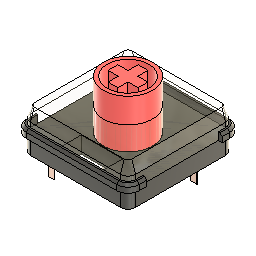
Choc v2 v34 (Autodesk Fusion 360 design; units mm, degrees)
Autodesk Fusion 360 part; units mm, degrees
note: some values were not read from the file. Chosen so that the rebuilt part matches the saved one: which face or edge a step refers to; a side; which pieces of a blend or face edit are solid. Set by a fixed rule: which sketch regions a step uses.
sketch "Base" plane through (0, 0, 0) normal (0, 0, 1) x (1, 0, 0)
  line L0 (6, 7.5) -> (-6, 7.5)
  line L1 (-7.5, 6) -> (-7.5, -6)
  line L2 (-6, -7.5) -> (6, -7.5)
  line L3 (7.5, -6) -> (7.5, 6)
  line L4 (7.5, 7.5) -> (-7.5, -7.5) construction
  line L5 (-7.5, 7.5) -> (7.5, -7.5) construction
  line L6 (-9, 5) -> (9, 5)
  line L7 (20, 0) -> (2.5, 0)
  line L8 (-9, -5) -> (9, -5)
  line L9 (5.975, 6.975) -> (-5.975, 6.975)
  line L10 (-6.975, 5.975) -> (-6.975, -5.975)
  line L11 (-5.975, -6.975) -> (5.975, -6.975)
  line L12 (6.975, -5.975) -> (6.975, 5.975)
  line L13 (6.975, 6.975) -> (-6.975, -6.975) construction
  line L14 (-6.975, 6.975) -> (6.975, -6.975) construction
  arc A0 (7.5, 6) -> (6, 7.5) centre (6, 6) ccw
  arc A1 (6, -7.5) -> (7.5, -6) centre (6, -6) ccw
  arc A2 (-7.5, -6) -> (-6, -7.5) centre (-6, -6) ccw
  arc A3 (-6, 7.5) -> (-7.5, 6) centre (-6, 6) ccw
  arc A4 (6.975, 5.975) -> (5.975, 6.975) centre (5.975, 5.975) ccw
  arc A5 (5.975, -6.975) -> (6.975, -5.975) centre (5.975, -5.975) ccw
  arc A6 (-6.975, -5.975) -> (-5.975, -6.975) centre (-5.975, -5.975) ccw
  arc A7 (-5.975, 6.975) -> (-6.975, 5.975) centre (-5.975, 5.975) ccw
  circle A8 centre (0, 0) radius 3.25
  circle A9 centre (0, 0) radius 2.4
  line L15 (2.75, -3.455) -> (-2.75, -3.455)
  line L16 (-2.75, -3.455) -> (-2.75, -6.405)
  line L17 (-2.75, -6.405) -> (2.75, -6.405)
  line L18 (2.75, -6.405) -> (2.75, -3.455)
  line L19 (2.75, -3.455) -> (-2.75, -6.405) construction
  line L20 (-2.75, -3.455) -> (2.75, -6.405) construction
  line L21 (0, 1.75) -> (0, 22.5)
  line L22 (2, 0.65) -> (-2, 0.65)
  line L23 (-2, 0.65) -> (-2, -0.65)
  line L24 (-2, -0.65) -> (2, -0.65)
  line L25 (2, -0.65) -> (2, 0.65)
  line L26 (2, 0.65) -> (-2, -0.65) construction
  line L27 (-2, 0.65) -> (2, -0.65) construction
  line L28 (0.65, 2) -> (0.65, -2)
  line L29 (-0.65, 2) -> (0.65, 2)
  line L30 (-0.65, -2) -> (-0.65, 2)
  line L31 (0.65, -2) -> (-0.65, -2)
  line L32 (-4.6, -5.1) -> (-5.4, -5.1)
  line L33 (-5.4, -5.1) -> (-5.4, -5.2)
  line L34 (-5.4, -5.2) -> (-4.6, -5.2)
  line L35 (-4.6, -5.2) -> (-4.6, -5.1)
  line L36 (-4.6, -5.1) -> (-5.4, -5.2) construction
  line L37 (-5.4, -5.1) -> (-4.6, -5.2) construction
  line L38 (1.75, 0) -> (22.5, 0)
  line L39 (0.4, 5.95) -> (-0.4, 5.95)
  line L40 (-0.4, 5.95) -> (-0.4, 5.85)
  line L41 (-0.4, 5.85) -> (0.4, 5.85)
  line L42 (0.4, 5.85) -> (0.4, 5.95)
  line L43 (0.4, 5.95) -> (-0.4, 5.85) construction
  line L44 (-0.4, 5.95) -> (0.4, 5.85) construction
  line L45 (5.4, 3.85) -> (4.6, 3.85)
  line L46 (4.6, 3.85) -> (4.6, 3.75)
  line L47 (4.6, 3.75) -> (5.4, 3.75)
  line L48 (5.4, 3.75) -> (5.4, 3.85)
  line L49 (5.4, 3.85) -> (4.6, 3.75) construction
  line L50 (4.6, 3.85) -> (5.4, 3.75) construction
  line L51 (9.9048, 2.5) -> (-9, 2.5)
  line L52 (9.9048, -2.5) -> (-9, -2.5)
  circle A10 centre (-5, -5.15) radius 0.7
  line L53 (-5, -5.85) -> (-3.3, -5.85)
  line L54 (-3.3, -5.85) -> (-3.3, -3.5282)
  line L55 (-3.3, -3.5282) -> (-5.7, -3.5282)
  line L56 (-5.7, -3.5282) -> (-5.7, -5.15)
  arc A11 (-5.7, -5.15) -> (-5, -5.85) centre (-5, -5.15) ccw
  line L57 (6, -7.5) -> (7.5, -7.5)
  line L58 (7.5, -6) -> (7.5, -7.5)
  line L59 (7.5, 6) -> (7.5, 7.5)
  line L60 (6, 7.5) -> (7.5, 7.5)
  line L61 (-6, 7.5) -> (-7.5, 7.5)
  line L62 (-7.5, 6) -> (-7.5, 7.5)
  line L63 (-7.5, -6) -> (-7.5, -7.5)
  line L64 (-6, -7.5) -> (-7.5, -7.5)
  line L65 (7.5, -2.5) -> (7.5, 2.5)
  line L66 (7.5, 2.5) -> (8.975, 2.5)
  line L67 (8.975, 2.5) -> (8.975, -2.5)
  line L68 (8.975, -2.5) -> (7.5, -2.5)
  line L69 (-7.5, -2.5) -> (-7.5, 2.5)
  line L70 (-7.5, 2.5) -> (-8.975, 2.5)
  line L71 (-8.975, 2.5) -> (-8.975, -2.5)
  line L72 (-8.975, -2.5) -> (-7.5, -2.5)
  point P0 (0, -4.93)
  point P1 (-5, -5.15)
  point P2 (0, 5.9)
  point P3 (5, 3.8)
  point P4 (-5, -5.15)
  dimension "d1" = 15
  dimension "d2" = 10
  dimension "d3" = 13.95
  dimension "d4" = 1.5
  dimension "d5" = 1
  dimension "d6" = 6.5
  dimension "d7" = 4.8
  dimension "d25" = 4.93
  dimension "d26" = 2.95
  dimension "d27" = 5.5
  dimension "d30" = 4
  dimension "d31" = 1.3
  dimension "d34" = 5.15
  dimension "d35" = 5
  dimension "d36" = 0.8
  dimension "d37" = 0.1
  dimension "d41" = 0.1
  dimension "d42" = 0.8
  dimension "d43" = 5.9
  dimension "d44" = 0.1
  dimension "d45" = 0.8
  dimension "d46" = 5
  dimension "d47" = 3.8
  dimension "d54" = 5
  dimension "d58" = 1.4
  dimension "d74" = 0.7
  dimension "d91" = 2
  dimension "d92" = 2
  constraint horizontal L0
  constraint perpendicular L0 L1
  constraint parallel L0 L2
  constraint parallel L1 L3
  constraint coincident L4 A8.centre
  constraint coincident L5 A8.centre
  constraint coincident A8.centre A9.centre
  constraint perpendicular L3 L6
  constraint symmetric L6.start L7 L8.start
  constraint symmetric L6.end L7 L8.end
  constraint horizontal L9
  constraint perpendicular L9 L10
  constraint parallel L9 L11
  constraint parallel L10 L12
  constraint coincident L4 L13.start
  constraint coincident L13 A8.centre
  constraint coincident L14 A8.centre
  constraint coincident L4.start L0
  constraint coincident L4.start L3
  constraint tangent L0 A0
  constraint tangent L3 A0
  constraint coincident L5.end L3
  constraint coincident L5.end L2
  constraint tangent L3 A1
  constraint tangent L2 A1
  constraint equal A0 A1
  constraint coincident L4.end L2
  constraint coincident L4.end L1
  constraint tangent L2 A2
  constraint tangent L1 A2
  constraint equal A0 A2
  constraint coincident L5.start L1
  constraint coincident L5.start L0
  constraint tangent L1 A3
  constraint tangent L0 A3
  constraint equal A0 A3
  constraint equal L0 L1
  constraint coincident L13.start L9
  constraint coincident L13.start L12
  constraint tangent L9 A4
  constraint tangent L12 A4
  constraint coincident L14.end L12
  constraint coincident L14.end L11
  constraint tangent L12 A5
  constraint tangent L11 A5
  constraint equal A4 A5
  constraint coincident L13.end L11
  constraint coincident L13.end L10
  constraint tangent L11 A6
  constraint tangent L10 A6
  constraint equal A4 A6
  constraint coincident L14.start L10
  constraint coincident L14.start L9
  constraint tangent L10 A7
  constraint tangent L9 A7
  constraint equal A4 A7
  constraint horizontal L15
  constraint perpendicular L15 L16
  constraint parallel L15 L17
  constraint parallel L16 L18
  constraint coincident L19 P0
  constraint coincident L20 P0
  constraint coincident P0 L21
  constraint horizontal L22
  constraint perpendicular L22 L23
  constraint parallel L22 L24
  constraint parallel L23 L25
  constraint coincident L26 A8.centre
  constraint coincident L27 A8.centre
  constraint symmetric L4 L22.start L28.start
  constraint symmetric L4 L22.end L28.end
  constraint symmetric L4 L23.end L30.start
  constraint symmetric L4 L24.end L29.start
  constraint horizontal L32
  constraint perpendicular L32 L33
  constraint parallel L32 L34
  constraint parallel L33 L35
  constraint coincident L36 P4
  constraint coincident L37 P4
  constraint horizontal L39
  constraint perpendicular L39 L40
  constraint parallel L39 L41
  constraint parallel L40 L42
  constraint coincident L43 P2
  constraint coincident L44 P2
  constraint coincident L21 P2
  constraint horizontal L45
  constraint perpendicular L45 L46
  constraint parallel L45 L47
  constraint parallel L46 L48
  constraint coincident L49 P3
  constraint coincident L50 P3
  constraint perpendicular L1 L51
  constraint symmetric L7 L51.start L52.start
  constraint symmetric L7 L51.end L52.end
  constraint coincident P4 P1
  constraint horizontal L53
  constraint perpendicular L53 L54
  constraint tangent L53 A11
  constraint tangent L56 A11
  constraint tangent A1 L57
  constraint tangent A0 L59
  constraint tangent A0 L60
  constraint perpendicular L65 L66
  constraint parallel L65 L67
  constraint parallel L66 L68
  constraint coincident L3 L65.end
  constraint coincident L51 L65.end
  constraint perpendicular L51 L65
  constraint coincident L52 L65.start
  constraint perpendicular L69 L70
  constraint parallel L69 L71
  constraint parallel L70 L72
  constraint coincident L1 L69.end
  constraint coincident L51 L69.end
  constraint perpendicular L51 L69
  constraint coincident L52 L69.start
  measures "d1" distance of L1 L3
  measures "d2" distance of L6 L8
  measures "d3" distance of L10 L12
  measures "d4" radius of A0
  measures "d5" radius of A4
  measures "d6" diameter of A8
  measures "d7" diameter of A9
  measures "d25" distance of A8.centre P0
  measures "d26" distance of L15 L17
  measures "d27" distance of L16 L18
  measures "d30" distance of L23 L25
  measures "d31" distance of L22 L24
  measures "d34" distance of P4 L38
  measures "d35" distance of L21 P4
  measures "d36" distance of L33 L35
  measures "d37" distance of L32 L34
  measures "d41" distance of L39 L41
  measures "d42" distance of L40 L42
  measures "d43" distance of A8.centre P2
  measures "d44" distance of L45 L47
  measures "d45" distance of L46 L48
  measures "d46" distance of L21 P3
  measures "d47" distance of L38 P3
  measures "d54" distance of L51 L52
  measures "d58" diameter of A10
  measures "d74" radius of A11
  measures "d91" distance of L12 L67
  measures "d92" distance of L10 L71
extrude "Extrude1" add sketch "Base" along normal blind 3.1 contours L6 L9 L10 A7 L21 L39 L40 L41 | L6 L9 L12 A4 L21 L39 L41 L42 | L21 L39 L41 L42 | L21 L39 L40 L41 | L6 L12 A8 L21 L51 | L7 L12 A8 L38 L51 | L6 L10 A8 L21 L51 | L7 L12 A8 L38 L52 | L10 A8 L51 L52 | L8 L10 L12 A8 L15 L16 L18 L52 L54 L55 L56 | L8 L10 L11 L12 A5 A6 L16 L17 L18 A10 L53 L54 L56 A11 | L8 L16 L17 L18 | L8 L15 L16 L18 | L8 A10 L54 L55 L56 | L8 A10 L56 | L8 A10 | L8 A10 A11 | L8 A10 L53 L54 | L32 L33 L34 L35 | L45 L46 L47 L48 makes body 1
chamfer "Chamfer1" distance 0.5 distance2 1.5 8 edges at (6.975, 0, 3.1) (6.6821, 6.6821, 3.1) (0, 6.975, 3.1) (-6.6821, 6.6821, 3.1) (-6.975, 0, 3.1) (-6.6821, -6.6821, 3.1) (0, -6.975, 3.1) (6.6821, -6.6821, 3.1) measured on face at (6.975, -1.6667, 1.0333) measured on face at (6.1643, 6.9569, 2.0667) measured on face at (3.9833, 6.975, 1.0333) measured on face at (-6.92, 6.3021, 2.0667) measured on face at (-6.975, 0.8333, 1.0333) measured on face at (-6.3021, -6.92, 2.0667) measured on face at (-1.9917, -6.975, 1.0333) measured on face at (6.9569, -6.1643, 2.0667) on bodies 1
extrude "Extrude2" add sketch "Base" along normal blind 1 separate body contours L0 L3 L6 L9 L12 A0 A4 L21 | L0 L1 L6 L9 L10 A3 A7 L21 | L1 L2 L3 L8 L10 L11 L12 A1 A2 A5 A6 makes body 2 at (2, 7.5, 0.3333) makes body 3 at (-2, -7.5, 0.3333)
chamfer "Chamfer2" distance 0.3 distance2 0.3 10 edges at (0, -7.5, 1) (7.0607, -7.0607, 1) (7.5, -5.5, 1) (-7.5, -5.5, 1) (-7.0607, -7.0607, 1) (0, 7.5, 1) (-7.0607, 7.0607, 1) (-7.5, 5.5, 1) (7.5, 5.5, 1) (7.0607, 7.0607, 1) measured on face at (1.9917, -7.325, 1) measured on face at (1.9917, -7.325, 1) measured on face at (1.9917, -7.325, 1) measured on face at (1.9917, -7.325, 1) measured on face at (1.9917, -7.325, 1) measured on face at (-1.9917, 7.325, 1) measured on face at (-1.9917, 7.325, 1) measured on face at (-1.9917, 7.325, 1) measured on face at (-1.9917, 7.325, 1) measured on face at (-1.9917, 7.325, 1) on bodies 2 3
extrude "Extrude3" add sketch "Base" against normal blind 2.2 separate body contours L6 L9 L10 A7 L21 L39 L40 L41 | L6 L9 L12 A4 L21 L39 L41 L42 | L21 L39 L41 L42 | L21 L39 L40 L41 | L6 L12 A8 L21 L51 | L7 L12 A8 L38 L51 | L6 L10 A8 L21 L51 | L7 L12 A8 L38 L52 | A8 L21 L51 | L7 A8 A9 L21 L38 L51 | A8 L21 L51 | L10 A8 L51 L52 | L8 L10 L12 A8 L15 L16 L18 L52 L54 L55 L56 | L7 A8 A9 L21 L38 L51 L52 | L8 L10 L11 L12 A5 A6 L16 L17 L18 A10 L53 L54 L56 A11 | A8 L52 | L8 L16 L17 L18 | L8 L15 L16 L18 | L8 A10 L54 L55 L56 | L8 A10 L56 | L8 A10 | L8 A10 A11 | L8 A10 L53 L54 | L32 L33 L34 L35 | L45 L46 L47 L48 makes body 4
extrude "Extrude4" add sketch "Base" along normal blind 6.4 thin wall 0.5 inside separate body contours A8 L21 L51 | L7 A8 A9 L21 L38 L51 | A8 L21 L51 | L7 A8 A9 L21 L38 L51 L52 | A8 L52 | A9 L21 L22 L23 L24 L25 L28 L29 L30 L31 L38 | A9 L21 L22 L25 L28 L29 L38 | L22 L28 L29 L30 | L22 L24 L25 L28 | L22 L23 L24 L30 | L22 L24 L28 L30 | L24 L28 L30 L31 makes body 5
extrude "Extrude5" add sketch "Base" against normal blind 5.5 separate body contours A9 L21 L22 L23 L24 L25 L28 L29 L30 L31 L38 | A9 L21 L22 L25 L28 L29 L38 | L22 L28 L29 L30 | L22 L24 L25 L28 | L22 L23 L24 L30 | L22 L24 L28 L30 | L24 L28 L30 L31 makes body 6
chamfer "Chamfer3" distance 0.5 distance2 0.8 1 edges at (-2.2376, 0.8679, -5.5) measured on face at (0.4722, 0.2704, -5.5) on bodies 6
extrude "Extrude6" cut sketch "Base" against normal up to surface (2.2 mm away) contours L8 L16 L17 L18 | L8 L15 L16 L18 bodies 4
extrude "Extrude7" add sketch "Base" along normal blind 6.4 separate body contours L22 L28 L29 L30 | L22 L24 L25 L28 | L22 L23 L24 L30 | L22 L24 L28 L30 | L24 L28 L30 L31 makes body 7
combine "Combine1" operation add target body 2 tool bodies 3 4 6
extrude "Extrude8" add sketch "Base" against normal blind 3 from surface at -2.2 separate body contours L32 L33 L34 L35 makes body 8
extrude "Extrude9" add sketch "Base" against normal blind 3 from surface at -2.2 separate body contours L21 L39 L41 L42 | L21 L39 L40 L41 | L45 L46 L47 L48 makes body 9 at (4.8667, 3.75, -4.2) makes body 10 at (0.1333, 5.95, -3.2)
extrude "Extrude10" add sketch "Base" against normal blind 2.25 separate body contours L6 L9 L10 A7 L21 L39 L40 L41 | L6 L9 L12 A4 L21 L39 L41 L42 | L21 L39 L41 L42 | L21 L39 L40 L41 | L6 L12 A8 L21 L51 | L7 L12 A8 L38 L51 | L6 L10 A8 L21 L51 | L7 L12 A8 L38 L52 | A8 L21 L51 | L7 A8 A9 L21 L38 L51 | A8 L21 L51 | L10 A8 L51 L52 | L8 L10 L12 A8 L15 L16 L18 L52 L54 L55 L56 | L7 A8 A9 L21 L38 L51 L52 | L8 L10 L11 L12 A5 A6 L16 L17 L18 A10 L53 L54 L56 A11 | A8 L52 | A9 L21 L22 L23 L24 L25 L28 L29 L30 L31 L38 | A9 L21 L22 L25 L28 L29 L38 | L8 L16 L17 L18 | L8 L15 L16 L18 | L22 L28 L29 L30 | L8 A10 L54 L55 L56 | L8 A10 L56 | L22 L24 L25 L28 | L8 A10 | L8 A10 A11 | L8 A10 L53 L54 | L22 L23 L24 L30 | L22 L24 L28 L30 | L24 L28 L30 L31 | L32 L33 L34 L35 | L45 L46 L47 L48 makes body 11
ref_plane "WorkPlane1" through (0, 0, -1.4) normal (0, 0, 1) x (1, 0, 0)
ref_plane "WorkPlane2" through (0, 0, -1.45) normal (0, 0, 1) x (1, 0, 0)
sketch "Hook1" plane through (0, 0, -1.4) normal (0, 0, 1) x (1, 0, 0)
  line L0 (6.65, 2.5) -> (6.65, -2.5)
  line L1 (0, 1.75) -> (0, 22.5)
  line L2 (-6.65, 2.5) -> (-6.65, -2.5)
  line L3 (6.65, 2.5) -> (7, 2.5)
  line L4 (7, 2.5) -> (7, -2.5)
  line L5 (7, -2.5) -> (6.65, -2.5)
  line L6 (-6.65, 2.5) -> (-7, 2.5)
  line L7 (-7, 2.5) -> (-7, -2.5)
  line L8 (-7, -2.5) -> (-6.65, -2.5)
  dimension "d55" = 13.3
  constraint vertical L0
  constraint symmetric L0.start L1 L2.start
  constraint symmetric L0.end L1 L2.end
  constraint perpendicular L0 L3
  constraint perpendicular L3 L4
  constraint perpendicular L4 L5
  constraint symmetric L1 L3.end L6.end
  constraint symmetric L1 L4.end L7.end
  measures "d55" distance of L0 L2
sketch "Hook2" plane through (0, 0, -1.45) normal (0, 0, 1) x (1, 0, 0)
  line L0 (7, 2.5) -> (7.5, 2.5)
  line L1 (7.5, 2.5) -> (7.5, -2.5)
  line L2 (7.5, -2.5) -> (7, -2.5)
  line L3 (7, -2.5) -> (7, 2.5)
  line L4 (0, 1.75) -> (0, 22.5)
  line L5 (-7, 2.5) -> (-7.5, 2.5)
  line L6 (-7.5, 2.5) -> (-7.5, -2.5)
  line L7 (-7.5, -2.5) -> (-7, -2.5)
  line L8 (-7, -2.5) -> (-7, 2.5)
  constraint horizontal L0
  constraint perpendicular L0 L1
  constraint perpendicular L1 L2
  constraint perpendicular L0 L3
  constraint symmetric L0.start L4 L5.start
  constraint symmetric L0.end L4 L5.end
  constraint symmetric L1.end L4 L6.end
  constraint symmetric L2.end L4 L7.end
loft "Loft1" cut profiles "Hook1", "Base" section 1 contours L0 L3 L4 L5 section 2 contours L3 L7 L12 L38 L51 L65 | L3 L7 L12 L38 L52 L65 bodies 11
loft "Loft2" cut profiles "Hook1", "Base" section 1 contours L2 L6 L7 L8 section 2 contours L1 L10 L51 L52 L69 bodies 11
loft "Loft3" cut profiles "Hook1", "Hook2" section 1 contours L0 L3 L4 L5 section 2 contours L0 L1 L2 L3 bodies 11
loft "Loft4" cut profiles "Hook1", "Hook2" section 1 contours L2 L6 L7 L8 section 2 contours L5 L6 L7 L8 bodies 11
extrude "Extrude11" add sketch "Base" against normal blind 1 separate body contours L0 L3 L6 L9 L12 A0 A4 L21 | L0 L1 L6 L9 L10 A3 A7 L21 | L1 L2 L3 L8 L10 L11 L12 A1 A2 A5 A6 makes body 12 at (2, 7.5, -0.3333) makes body 13 at (-2, -7.5, -0.3333)
move_face "OffsetFaces6" offset -0.15 10 faces at (-7.5, 5.6667, -0.3333) (-7.4983, 6.0714, -0.6667) (2, 7.5, -0.3333) (6.4906, 7.4175, -0.6667) (7.5, 5.3333, -0.6667) (-2, -7.5, -0.3333) (6.5575, -7.3926, -0.6667) (7.5, -5.6667, -0.3333) (-6.6873, -7.3333, -0.6667) (-7.5, -5.3333, -0.3333) on bodies 12 13
copy_body "CopyPasteBodies1" bodies 1 makes body 14
combine "Combine2" operation add target body 14 tool bodies 2 keep tools
extrude "Extrude12" add sketch "Base" against normal blind 5 from surface at -2.2 separate body contours L8 A10 L54 L55 L56 | L8 A10 | L8 A10 A11 | L8 A10 L53 L54 | L32 L33 L34 L35 makes body 15
combine "Combine3" operation add target body 11 tool bodies 15
combine "Combine4" operation add target body 14 tool bodies 8 keep tools
sketch "Fill" plane through (0, 0, 0) normal (0, 0, 1) x (1, 0, 0)
  line L0 (11, -12) -> (-11, -12)
  line L1 (-12, -11) -> (-12, 11)
  line L2 (-11, 12) -> (11, 12)
  line L3 (12, 11) -> (12, -11)
  line L4 (12, -12) -> (-12, 12) construction
  line L5 (-12, -12) -> (12, 12) construction
  arc A0 (12, 11) -> (11, 12) centre (11, 11) ccw
  arc A1 (11, -12) -> (12, -11) centre (11, -11) ccw
  arc A2 (-12, -11) -> (-11, -12) centre (-11, -11) ccw
  arc A3 (-11, 12) -> (-12, 11) centre (-11, 11) ccw
  line L6 (8.5, -9.5) -> (-8.5, -9.5)
  line L7 (-9.5, -8.5) -> (-9.5, 8.5)
  line L8 (-8.5, 9.5) -> (8.5, 9.5)
  line L9 (9.5, 8.5) -> (9.5, -8.5)
  line L10 (9.5, -9.5) -> (-9.5, 9.5) construction
  line L11 (-9.5, -9.5) -> (9.5, 9.5) construction
  arc A4 (-8.5, 9.5) -> (-9.5, 8.5) centre (-8.5, 8.5) ccw
  arc A5 (-9.5, -8.5) -> (-8.5, -9.5) centre (-8.5, -8.5) ccw
  arc A6 (8.5, -9.5) -> (9.5, -8.5) centre (8.5, -8.5) ccw
  arc A7 (9.5, 8.5) -> (8.5, 9.5) centre (8.5, 8.5) ccw
  point P0 (-5.7422, -13.1336)
  point P1 (13.2578, -13.1336)
  point P2 (15.4591, -2.2153)
  point P3 (15.4591, -6.2153)
  dimension "d62" = 24
  dimension "Pitch" = 19
  dimension "BridgeR" = 1
  dimension "d66" = 24
  dimension "PitchMargin" = 4
  dimension "d83" = 19
  dimension "d84" = 1
  constraint horizontal L0
  constraint perpendicular L0 L1
  constraint parallel L0 L2
  constraint parallel L1 L3
  constraint coincident L4 origin
  constraint coincident L5 origin
  constraint coincident L5.end L2
  constraint coincident L5.end L3
  constraint tangent L2 A0
  constraint tangent L3 A0
  constraint coincident L4.start L3
  constraint coincident L4.start L0
  constraint tangent L3 A1
  constraint tangent L0 A1
  constraint equal A0 A1
  constraint coincident L5.start L0
  constraint coincident L5.start L1
  constraint tangent L0 A2
  constraint tangent L1 A2
  constraint equal A0 A2
  constraint coincident L4.end L1
  constraint coincident L4.end L2
  constraint tangent L1 A3
  constraint tangent L2 A3
  constraint equal A0 A3
  constraint horizontal L6
  constraint perpendicular L6 L7
  constraint parallel L6 L8
  constraint parallel L7 L9
  constraint coincident L4 L10.start
  constraint coincident L10 origin
  constraint coincident L11 origin
  constraint coincident L10.end L8
  constraint coincident L10.end L7
  constraint tangent L8 A4
  constraint tangent L7 A4
  constraint coincident L11.start L7
  constraint coincident L11.start L6
  constraint tangent L7 A5
  constraint tangent L6 A5
  constraint equal A4 A5
  constraint coincident L10.start L6
  constraint coincident L10.start L9
  constraint tangent L6 A6
  constraint tangent L9 A6
  constraint equal A4 A6
  constraint coincident L11.end L9
  constraint coincident L11.end L8
  constraint tangent L9 A7
  constraint tangent L8 A7
  constraint equal A4 A7
  measures "d62" distance of L1 L3
  measures "Pitch" distance of P0 P1
  measures "BridgeR" radius of A0
  measures "d66" distance of L0 L2
  measures "PitchMargin" distance of P2 P3
  measures "d83" distance of L10.end L11.end
  measures "d84" radius of A4
extrude "Extrude13" add sketch "Fill" against normal blind 5.5 separate body contours L0 L1 L2 L3 A0 A1 A2 A3 | L6 L7 L8 L9 A4 A5 A6 A7 makes body 16
extrude "Extrude14" add sketch "Base" along normal blind 10 separate body contours L0 L3 L6 L9 L12 A0 A4 L21 | A0 L59 L60 | L0 L1 L6 L9 L10 A3 A7 L21 | A3 L61 L62 | L6 L9 L10 A7 L21 L39 L40 L41 | L6 L9 L12 A4 L21 L39 L41 L42 | L3 L6 L12 L51 | L21 L39 L41 L42 | L21 L39 L40 L41 | L3 L7 L12 L38 L51 L65 | L6 L12 A8 L21 L51 | L1 L6 L10 L51 | L3 L7 L12 L38 L52 L65 | L7 L12 A8 L38 L51 | L6 L10 A8 L21 L51 | L1 L10 L51 L52 L69 | L3 L8 L12 L52 | L7 L12 A8 L38 L52 | A8 L21 L51 | L7 A8 A9 L21 L38 L51 | A8 L21 L51 | L1 L8 L10 L52 | L10 A8 L51 L52 | L1 L2 L3 L8 L10 L11 L12 A1 A2 A5 A6 | L8 L10 L12 A8 L15 L16 L18 L52 L54 L55 L56 | L7 A8 A9 L21 L38 L51 L52 | A1 L57 L58 | L8 L10 L11 L12 A5 A6 L16 L17 L18 A10 L53 L54 L56 A11 | A8 L52 | A9 L21 L22 L23 L24 L25 L28 L29 L30 L31 L38 | A9 L21 L22 L25 L28 L29 L38 | A2 L63 L64 | L8 L16 L17 L18 | L8 L15 L16 L18 | L22 L28 L29 L30 | L8 A10 L54 L55 L56 | L8 A10 L56 | L22 L24 L25 L28 | L8 A10 | L8 A10 A11 | L8 A10 L53 L54 | L22 L23 L24 L30 | L22 L24 L28 L30 | L24 L28 L30 L31 | L32 L33 L34 L35 | L45 L46 L47 L48 makes body 17
move_face "OffsetFaces2" offset 0.5 3 faces at (-6.5, -7.5, 3.3333) (-2, -7.5, 3.3333) (6.5, -7.5, 3.3333) on bodies 17
move_face "OffsetFaces3" offset 0.5 8 faces at (7.5, -1.6667, 3.3333) (7.5, 0.8333, 3.3333) (7.5, -4.1667, 3.3333) (7.5, -5.6667, 3.3333) (7.5, -6.6667, 6.6667) (7.5, 7, 6.6667) (7.5, 5.3333, 3.3333) (7.5, 3.3333, 3.3333) on bodies 17
move_face "OffsetFaces4" offset 0.5 4 faces at (-6.5, 7.5, 3.3333) (-2, 7.5, 3.3333) (4, 7.5, 3.3333) (6.6667, 7.5, 6.6667) on bodies 17
move_face "OffsetFaces5" offset 0.5 7 faces at (-7.5, -6.6667, 3.3333) (-7.5, -5.3333, 3.3333) (-7.5, -3.3333, 3.3333) (-7.5, 0.8333, 3.3333) (-7.5, 4.1667, 3.3333) (-7.5, 5.6667, 3.3333) (-7.5, 6.6667, 3.3333) on bodies 17
extrude "Extrude15" add sketch "Base" along normal up to surface (10 mm away) and the other way blind 0.8 contours L3 L7 L38 L51 L65 L66 L67 | L3 L7 L12 L38 L51 L65 | L3 L7 L38 L52 L65 L67 L68 | L3 L7 L12 L38 L52 L65 | L7 L12 A8 L38 L51 | L1 L10 L51 L52 L69 | L1 L51 L52 L69 L70 L71 L72 | L7 L12 A8 L38 L52 | L7 A8 A9 L21 L38 L51 | L10 A8 L51 L52 | L7 A8 A9 L21 L38 L51 L52 | A9 L21 L22 L23 L24 L25 L28 L29 L30 L31 L38 | A9 L21 L22 L25 L28 L29 L38 | L22 L28 L29 L30 | L22 L24 L25 L28 | L22 L23 L24 L30 | L22 L24 L28 L30 | L24 L28 L30 L31 bodies 17
fillet "Fillet1" radius 0.3 12 edges at (-8, 8, 5) (8, 8, 5) (-8, -8, 5) (8, -8, 5) (-8, -2.5, 5) (-8, 2.5, 5) (8.975, -2.5, 4.6) (8, -2.5, 5) (8.975, 2.5, 4.6) (8, 2.5, 5) (-8.975, -2.5, 4.6) (-8.975, 2.5, 4.6) on bodies 17
combine "Combine6" operation add target body 11 tool bodies 17
chamfer "Chamfer4" distance 0.3 angle 45 10 edges at (-7.35, 5.5, -1) (-6.9546, 6.9546, -1) (0, 7.35, -1) (6.9546, 6.9546, -1) (7.35, 5.5, -1) (0, -7.35, -1) (6.9546, -6.9546, -1) (7.35, -5.5, -1) (-7.35, -5.5, -1) (-6.9546, -6.9546, -1) on bodies 12 13
copy_body "CopyPasteBodies3" bodies 16 makes body 18
combine "Combine7" operation add target body 18 tool bodies 11 keep tools
hidden bodies 11 12 13 14 16 18
equation "d62 = Pitch + BridgeR + PitchMargin"
equation "d66 = Pitch + BridgeR + PitchMargin"
equation "d83 = Pitch"
equation "d84 = BridgeR"
named bodies: "Hole", "MF", "Fill", "Territory", "MF2"
